side_long_v18 (Autodesk Fusion 360 design; units mm, degrees)
Autodesk Fusion 360 part; units mm, degrees
sketch "Sketch1" plane through (0, 0, 0) normal (0, 0, 1) x (1, 0, 0)
  line L0 (0, 0) -> (433.8, 0)
  line L1 (433.8, 0) -> (433.8, 70.4)
  line L2 (433.8, 70.4) -> (0, 70.4)
  line L3 (0, 70.4) -> (0, 0)
  line L4 (0, 0) -> (19.9, 0)
  line L5 (19.9, 0) -> (19.9, 32.4)
  line L6 (19.9, 32.4) -> (0, 32.4)
  line L7 (0, 32.4) -> (0, 0)
  line L8 (206.95, 0) -> (226.85, 0)
  line L9 (226.85, 0) -> (226.85, 32.4)
  line L10 (226.85, 32.4) -> (206.95, 32.4)
  line L11 (206.95, 32.4) -> (206.95, 0)
  line L12 (433.8, 0) -> (413.9, 0)
  line L13 (413.9, 0) -> (413.9, 32.4)
  line L14 (413.9, 32.4) -> (433.8, 32.4)
  line L15 (433.8, 32.4) -> (433.8, 0)
  dimension "d1" = 433.8
  dimension "d2" = 70.4
  dimension "d3" = 19.9
  dimension "d4" = 19.9
  dimension "d5" = 19.9
  dimension "d6" = 32.4
  dimension "d7" = 32.4
  dimension "d8" = 32.4
  dimension "d9" = 206.95
  constraint horizontal L0
  constraint vertical L1
  constraint horizontal L2
  constraint vertical L3
  constraint coincident L0.start L3.end
  constraint horizontal L4
  constraint vertical L5
  constraint horizontal L6
  constraint vertical L7
  constraint coincident L0 L3.end
  constraint horizontal L8
  constraint vertical L9
  constraint horizontal L10
  constraint vertical L11
  constraint coincident L0 L8.start
  constraint horizontal L12
  constraint vertical L13
  constraint horizontal L14
  constraint vertical L15
  measures "d1" distance of L0.start L0.end
  measures "d2" distance of L0.start L2.end
  measures "d3" distance of L5.end L6.end
  measures "d4" distance of L9.end L10.end
  measures "d5" distance of L13.end L14.end
  measures "d6" distance of L0 L6
  measures "d7" distance of L8.start L10.end
  measures "d8" distance of L12.end L13.end
  measures "d9" distance of L1 L9
extrude "Extrude2" add sketch "Sketch1" along normal blind 5.4 contours L0 L1 L2 L3 L5 L6 L9 L10 L11 L13 L14
sketch "Sketch2" plane through (0, 0, 5.4) normal (0, 0, 1) x (1, 0, 0)
  line L0 (226.85, 0) -> (413.9, 0)
  line L1 (413.9, 0) -> (413.9, 32.4)
  line L2 (413.9, 32.4) -> (433.8, 32.4)
  line L3 (433.8, 32.4) -> (433.8, 70.4)
  line L4 (433.8, 70.4) -> (0, 70.4)
  line L5 (0, 70.4) -> (0, 32.4)
  line L6 (0, 32.4) -> (19.9, 32.4)
  line L7 (19.9, 32.4) -> (19.9, 0)
  line L8 (19.9, 0) -> (206.95, 0)
  line L9 (206.95, 0) -> (206.95, 32.4)
  line L10 (206.95, 32.4) -> (226.85, 32.4)
  line L11 (226.85, 32.4) -> (226.85, 0)
  line L12 (256.9, 32.4) -> (176.9, 32.4)
  arc A0 (176.9, 32.4) -> (176.9, 22.4) centre (176.9, 27.4) ccw
  line L13 (176.9, 22.4) -> (256.9, 22.4)
  arc A1 (256.9, 22.4) -> (256.9, 32.4) centre (256.9, 27.4) ccw
  line L14 (256.9, 27.4) -> (176.9, 27.4) construction
  point P0 (216.9, 27.4)
  dimension "d14" = 5
  dimension "d15" = 80
  dimension "d16" = 433.8
  dimension "d17" = 216.9
  constraint tangent L12 A0
  constraint tangent A0 L13
  constraint parallel L12 L13
  constraint tangent L13 A1
  constraint tangent L12 A1
  constraint horizontal L14
  constraint midpoint L14 P0
  constraint collinear L10 L12
  measures "d14" radius of A0
  measures "d15" distance of A1.centre A0.centre
  measures "d16" distance of L3.end L4.end
  measures "d17" distance of L5 P0
extrude "Extrude3" cut sketch "Sketch2" against normal blind 25 contours L11 L12 L13 A1 | L9 L12 A0 L13
sketch "export" plane through (0, 0, 5.4) normal (0, 0, 1) x (1, 0, 0)
  line L0 (206.95, 22.4) -> (176.9, 22.4)
  arc A0 (176.9, 32.4) -> (176.9, 22.4) centre (176.9, 27.4) ccw
  line L1 (176.9, 32.4) -> (256.9, 32.4)
  arc A1 (256.9, 22.4) -> (256.9, 32.4) centre (256.9, 27.4) ccw
  line L2 (256.9, 22.4) -> (226.85, 22.4)
  line L3 (226.85, 22.4) -> (226.85, 0)
  line L4 (226.85, 0) -> (413.9, 0)
  line L5 (413.9, 0) -> (413.9, 32.4)
  line L6 (413.9, 32.4) -> (433.8, 32.4)
  line L7 (433.8, 32.4) -> (433.8, 70.4)
  line L8 (433.8, 70.4) -> (0, 70.4)
  line L9 (0, 70.4) -> (0, 32.4)
  line L10 (0, 32.4) -> (19.9, 32.4)
  line L11 (19.9, 32.4) -> (19.9, 0)
  line L12 (19.9, 0) -> (206.95, 0)
  line L13 (206.95, 0) -> (206.95, 22.4)
extrude "Extrude1" [suppressed]
equation "d2 = d6 + 38 mm"
equation "d4 = d3"
equation "d5 = d4"
equation "d6 = 6 * 5.4 mm"
equation "d7 = d6"
equation "d8 = d7"
equation "d9 = ( d1 - d4 ) / 2"
equation "d17 = d16 / 2"
